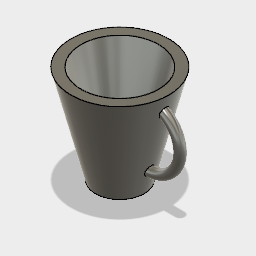
cup (Autodesk Fusion 360 design; units mm, degrees)
Autodesk Fusion 360 part; units mm, degrees
note: some values were not read from the file. Set by a fixed rule: which face or edge a step refers to.
cylinder "圆柱体基本要素1" add diameter 20 height 20 placed x (1, 0, 0) y (0, 0, -1) z (0, 1, 0) at (0, 0, 0)
sketch "草图4" plane through (0, 0, 0) normal (0, -1, 0) x (1, 0, 0)
  circle A0 centre (0, 0) radius 10
  circle A1 centre (0, 0) radius 5
loft "放样1" cut profiles "草图4" section 1 contours A1 section 2 face at (2.3712, 20, 3.5556) keep common part
torus "圆环体基本要素3" add centre line diameter 12.649 section diameter 2 placed x (1, 0, 0) y (0, 1, 0) z (0, 0, 1) at (6, 11, 0)
shell "抽壳1" thickness 2 removed faces 1 at (2.3712, 20, 3.5556)
torusprimitive "圆环体基本要素2" [suppressed]
